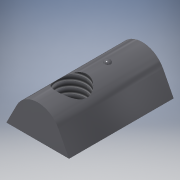
# Autodesk Inventor part: 20-058
Saved by Autodesk Inventor 2018 (Build 220105000, 105)
## iProperties
Created: 2004-10-14
Part Number: 20-058
Material: Steel, High Strength Low Alloy
Document SubType Name: Modeling
Designer: Autodesk, Inc.
Manufacturer: Standard
Standards Organization: Custom
Description: NUT, T SLOT, STANDARD, 40 SERIES, M8
Catalog Web Link: http://www.parker.com/ead/cm1.asp?cmid=809
Vendor: PARKER IPS
Mass: 10.738 g
Surface Area: 10.2004 cm^2
Volume: 1.36964 cm^3
Density: 7.84 g/cm^3
Appearance: Metal-Steel (Polished)
CAGE: 1LJX3
Dept. ID: Product Design
Description #2: ---
Finish #1: ---
Finish #2: ---
Material ID: ---
Project Number: ---
Author: Autodesk, Inc.
Autodesk Inventor part; units mm, degrees
ref_plane "YZ Plane" through (0, 0, 0) normal (1, 0, 0) x (0, 1, 0)
sketch "Sketch2" plane through (0, 0, 0) normal (0, 1, 0) x (-1, 0, 0)
  line L0 (6.9, -11.5) -> (-6.9, -11.5)
  line L1 (-6.9, -11.5) -> (-6.9, 11.5)
  line L2 (-6.9, 11.5) -> (6.9, 11.5)
  line L3 (6.9, 11.5) -> (6.9, -11.5)
  point P0 (0, 4)
  point P1 (0, -11.5)
  point P2 (0, 11.5)
  point P3 (0, 0)
  point P4 (-6.9, 0)
  dimension "CenterHole" = 7.5
  dimension "Length" = 23
  dimension "Width" = 13.8
  constraints: 8 end point, 3 midpoint, 2 parallel, 2 vertical alignment, 1 horizontal, 1 horizontal alignment, 1 perpendicular
  measures "CenterHole" distance from line of point (0, 4) L2
  measures "Length" distance of L2.end L0.start
  measures "Width" distance of L1.end L2.end
extrude "NutBase" add sketch "Sketch2" against normal blind 7.3
hole "Hole1" at (0, 0, 4) direction (0, -1, 0) diameter 6.647 end through all thread size "M8x1.25" class "6H" standard "ANSI Metric M Profile"
ref_plane "MidPlane" through (-6.9, 0, 0) normal (0, 0, -1) x (-1, 0, 0)
ref_plane "Work Plane4" through (6.9, 0, -3.8333) normal (0, 0, -1) x (-1, 0, 0)
sketch "Sketch3" plane through (-6.9, 0, 11.5) normal (0, 0, 1) x (1, 0, 0)
  line L0 (0, -7.3) -> (13.8, -7.3) construction
  line L1 (13.8, 0) -> (0, 0) projected
  line L2 (0, 0) -> (2.3, -4.4884)
  arc A0 (2.3, -4.4884) -> (11.5, -4.4884) centre (6.9, -2.1312) ccw
  line L3 (11.5, -4.4884) -> (13.8, 0)
  line L4 (6.9, -2.1312) -> (6.9, 0) construction
  dimension "d12" = 9.2
  constraints: 6 end point, 3 tangent, 2 point on circle, 1 centre point, 1 midpoint, 1 vertical
  measures "d12" distance of L3.start L2.end
extrude "Standard TSlot" cut sketch "Sketch3" along normal through all both and the other way through all keep common part
sketch "Sketch5" plane through (-6.9, 0, 11.5) normal (0, 0, 1) x (1, 0, 0)
  line L0 (0, -7.3) -> (13.8, -7.3) construction
  line L1 (13.8, 0) -> (0, 0) projected
  line L2 (0, 0) -> (0, -7.3) construction
  line L3 (6.9, 0) -> (6.9, -7.3) construction
  line L4 (0, -0.8) -> (2.95, -0.8)
  line L5 (2.95, -0.8) -> (2.95, 0)
  line L6 (2.95, 0) -> (0, 0)
  line L7 (0, 0) -> (0, -0.8)
  line L8 (13.8, -0.8) -> (10.85, -0.8)
  line L9 (10.85, -0.8) -> (10.85, 0)
  line L10 (10.85, 0) -> (13.8, 0)
  line L11 (13.8, 0) -> (13.8, -0.8)
  dimension "Slot_Width" = 7.9
  dimension "d18" = 0.8
  constraints: 18 end point, 5 symmetric about line, 2 midpoint, 2 parallel, 2 point on line, 1 horizontal, 1 perpendicular
  measures "Slot_Width" diameter of L5 L3
  measures "d18" distance between parallel lines of L1 L4
extrude "Self-Align TSlot" [suppressed]
sketch "Sketch6" plane through (-6.9, 0, 11.5) normal (0, 0, 1) x (1, 0, 0)
  line L0 (0, -7.3) -> (13.8, -7.3) projected
  line L1 (13.8, 0) -> (13.8, -7.3) projected
  line L2 (13.8, 0) -> (0, 0) projected
  line L3 (0, 0) -> (0, -7.3) projected
  line L4 (6.9, 0) -> (6.9, -7.3) construction
  line L5 (0, 0) -> (2.95, 0)
  line L6 (2.95, 0) -> (2.95, -3.5)
  line L7 (2.95, -3.5) -> (0, -3.5)
  line L8 (0, -3.5) -> (0, 0)
  line L9 (13.8, 0) -> (10.85, 0)
  line L10 (10.85, 0) -> (10.85, -3.5)
  line L11 (10.85, -3.5) -> (13.8, -3.5)
  line L12 (13.8, -3.5) -> (13.8, 0)
  arc A0 (0, -4.8) -> (2.5, -7.3) centre (2.5, -4.8) ccw
  arc A1 (11.3, -7.3) -> (13.8, -4.8) centre (11.3, -4.8) ccw
  dimension "HD_Slot_Depth" = 3.5
  dimension "HD_Slot_Width" = 7.9
  dimension "d23" = 2.5
  constraints: 18 end point, 4 point on circle, 4 point on line, 4 tangent, 3 symmetric about line, 2 centre point, 2 midpoint, 2 parallel, 1 horizontal, 1 perpendicular, 1 other
  measures "HD_Slot_Depth" distance of L7.end L2.end
  measures "HD_Slot_Width" diameter of L6 L4
  measures "d23" radius of A0
extrude "Heavy Duty TSlot" [suppressed]
sketch "Sketch7" plane through (0, 0, 0) normal (0, 1, 0) x (1, 0, 0)
  line L0 (-6.9, 11.5) -> (6.9, 11.5) projected
  line L1 (-6.9, -11.5) -> (-6.9, 11.5) projected
  line L2 (6.9, -11.5) -> (-6.9, -11.5) projected
  line L3 (6.9, 11.5) -> (6.9, -11.5) projected
  arc A0 (6.9, 8.7381) -> (-6.9, 8.7381) centre (0, 1.5) ccw
  arc A1 (-6.9, -8.7381) -> (6.9, -8.7381) centre (0, -1.5) ccw
  line L4 (-9.66, 0) -> (9.66, 0) construction
  point P0 (0, 11.5)
  point P1 (0, -11.5)
  dimension "Economy_Fillet_Size" = 10
  constraints: 6 point on circle, 4 point on line, 2 centre point, 2 horizontal alignment, 2 midpoint, 2 tangent, 1 other
  measures "Economy_Fillet_Size" radius of A0
extrude "Economy TSlot" [suppressed]
sketch "Sketch9" plane through (0, -7.3, 0) normal (0, -1, 0) x (1, 0, 0)
  arc A0 (8, 8.5) -> (-8, 8.5) centre (0, 2.5) ccw projected
  line L0 (-9.5459, -8.5) -> (-9.5459, 8.5) projected
  arc A1 (-8, -8.5) -> (8, -8.5) centre (0, -2.5) ccw projected
  line L1 (9.5459, 8.5) -> (9.5459, -8.5) projected
  circle A2 centre (0, 4) radius 3.3235 construction
  circle A3 centre (0, 4) radius 4.5735
  dimension "d35" = 1.25
  constraints: 1 centre point, 1 coincident
  measures "d35" radial gap between concentric circles of A2 A3
extrude "Economy TSlot2" [suppressed]
sketch "Sketch4" plane through (6.9, 0, -3.8333) normal (0, 0, -1) x (-1, 0, 0)
  circle A0 centre (6.9, -7.05) radius 0.75
  line L0 (6.9276, -6.3005) -> (6.8724, -6.3005)
  line L1 (6.9, -9.36) -> (6.9, 1.56) construction
  line L2 (13.8, -7.3) -> (0, -7.3) construction
  line L3 (6.9, -6.3005) -> (6.9, -7.8)
  line L4 (0, 0) -> (13.8, 0) construction
  dimension "d15" = 1.5
  dimension "d38" = 7.05
  constraints: 4 end point, 3 point on circle, 3 point on line, 1 centre point, 1 midpoint
  measures "d15" diameter of A0
  measures "d38" distance from line of L4 A0.centre
revolve "SpringBall" add sketch "Sketch4" angle 360 about axis through (0, -10, -3.8333) along (0, 1, 0) picked at (6.8409, -7.2931) contours A0 L3
mirror "Double Mirror" [suppressed]
sketch "Sketch10" plane through (-6.9, 0, 11.5) normal (0, 0, 1) x (1, 0, 0)
  line L0 (6.9, -8.76) -> (6.9, 1.46) construction
  line L1 (0, 0) -> (4.0362, 0)
  line L2 (4.0362, 0) -> (4.0362, -1.925)
  line L3 (4.0362, -1.925) -> (0, -1.925)
  line L4 (0, -1.925) -> (0, 0)
  line L5 (13.8, 0) -> (9.7638, 0)
  line L6 (9.7638, 0) -> (9.7638, -1.925)
  line L7 (9.7638, -1.925) -> (13.8, -1.925)
  line L8 (13.8, -1.925) -> (13.8, 0)
  dimension "d40" = 5.7276
  dimension "d41" = 1.925
  constraints: 16 end point, 3 symmetric about line, 2 parallel, 1 horizontal, 1 perpendicular
  measures "d40" distance between parallel lines of L6 L2
  measures "d41" distance between parallel lines of L1 L3
extrude "Zn TSlot 1" [suppressed]
sketch "Sketch11" plane through (0, -7.3, 0) normal (0, -1, 0) x (1, 0, 0)
  circle A0 centre (0, 4) radius 3.3235 projected
  line L0 (-6.9, -11.5) -> (-6.9, 11.5) projected
  line L1 (6.9, -11.5) -> (-6.9, -11.5) projected
  line L2 (6.9, -11.5) -> (-6.9, 2.3)
  line L3 (0, 4) -> (-6.9, 10.9) construction
  line L4 (6.9, 11.5) -> (6.9, -11.5) projected
  line L5 (-6.9, 11.5) -> (6.9, -2.3)
  line L6 (-6.9, 11.5) -> (6.9, 11.5) projected
  dimension "d44" = 45
  dimension "d45" = 12.1622
  dimension "d48" = 45
  constraints: 6 end point, 3 point on line, 2 coincident, 2 parallel
  measures "d44" angle of L1 L2
  measures "d45" diameter of L2 L3
  measures "d48" angle of L6 L5
extrude "Zn TSlot 2" [suppressed]
equation "\"d12\" = 0.666667 * Width"
equation "\"HD_Slot_Width\" = Slot_Width"
equation "\"d40\" = 0.707107 * Zn_C"
equation "\"d41\" = 0.25 * Zn_E"
equation "\"SpringBallPos\" = -0.333333 * Length"
equation "\"Zn_B\" = 27"
equation "\"Zn_C\" = 8.1"
equation "\"Zn_D\" = 7.9"
equation "\"Zn_E\" = 7.7"
body "Solid1"
